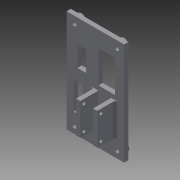
# Autodesk Inventor part: holder_board_basecam_simpleBCG_32bit_tiny
Saved by Autodesk Inventor 2015 SP1 (Build 190203100, 203)
## iProperties
Created: 2015-08-27
Part Number: holder_board_basecam_simpleBCG_32bit_tiny
Material: Generic
Document SubType Name: Modeling
Designer: Alexandre Cherpillod
Density: 1 g/cm^3
Appearance: Default
Author: Alexandre Cherpillod
Autodesk Inventor part; units mm, degrees
ref_plane "YZ Plane" through (0, 0, 0) normal (1, 0, 0) x (0, 1, 0)
ref_plane "XZ Plane" through (0, 0, 0) normal (0, 1, 0) x (-1, 0, 0)
ref_plane "XY Plane" through (0, 0, 0) normal (0, 0, 1) x (1, 0, 0)
sketch "Sketch1" plane through (0, 0, 0) normal (0, 1, 0) x (-1, 0, 0)
  circle A0 centre (0, 0) radius 2.4
  circle A1 centre (20, 0) radius 2.4
  circle A2 centre (20, -41.5) radius 2.4
  circle A3 centre (0, -41.5) radius 2.4
  dimension "d0" = 4.8
  dimension "d4" = 20
  dimension "d5" = 41.5
  constraints: 4 centre point, 3 equal radius, 1 coincident
  measures "d0" diameter of A0
  measures "d4" distance of point (0, 0) A1.centre
  measures "d5" distance of A2.centre A1.centre
extrude "Extrusion1" add sketch "Sketch1" along normal blind 1.5
sketch "Sketch2" plane through (0, 0, 0) normal (0, -1, 0) x (1, 0, 0)
  circle A0 centre (0, 0) radius 2.4 construction
  circle A1 centre (0, -41.5) radius 2.4 construction
  circle A2 centre (-20, -41.5) radius 2.4 construction
  circle A3 centre (-20, 0) radius 2.4 construction
  line L0 (3.492, 3.2394) -> (-23.508, 3.2394)
  line L1 (-23.508, 3.2394) -> (-23.508, -44.7606)
  line L2 (-23.508, -44.7606) -> (3.492, -44.7606)
  line L3 (3.492, -44.7606) -> (3.492, 3.2394)
  dimension "d8" = 27
  dimension "d9" = 48
  constraints: 8 end point, 2 parallel, 1 horizontal, 1 perpendicular
  measures "d8" distance of L0.start L0.end
  measures "d9" distance of L2.end L0.start
extrude "Extrusion2" add sketch "Sketch2" along normal blind 2
sketch "Sketch3" plane through (0, -2, 0) normal (0, -1, 0) x (1, 0, 0)
  circle A0 centre (0, 0) radius 2.4 construction
  circle A1 centre (0, -41.5) radius 2.4 construction
  circle A2 centre (-20, -41.5) radius 2.4 construction
  circle A3 centre (-20, 0) radius 2.4 construction
  line L0 (-8.5471, -21.5) -> (-10.5471, -21.5)
  line L1 (-10.5471, -21.5) -> (-10.5471, -36.5)
  line L2 (-10.5471, -36.5) -> (-8.5471, -36.5)
  line L3 (-8.5471, -36.5) -> (-8.5471, -21.5)
  line L4 (-0.5471, -21.5) -> (-2.5471, -21.5)
  line L5 (-2.5471, -21.5) -> (-2.5471, -36.5)
  line L6 (-2.5471, -36.5) -> (-0.5471, -36.5)
  line L7 (-0.5471, -36.5) -> (-0.5471, -21.5)
  line L8 (0, 0) -> (0, -41.5) construction
  dimension "d12" = 2
  dimension "d13" = 2
  dimension "d14" = 15
  dimension "d15" = 6
  dimension "d17" = 5
  constraints: 18 end point, 5 parallel, 2 horizontal, 2 perpendicular, 1 point on line, 1 vertical
  measures "d12" distance of L2.end L1.end
  measures "d13" distance of L6.end L5.end
  measures "d14" distance of L6.end L4.start
  measures "d15" distance between parallel lines of L3 L5
  measures "d17" distance from line of L8.end L6
extrude "Extrusion3" add sketch "Sketch3" along normal blind 8.5
sketch "Sketch4" plane through (-10.5471, -2, -36.5) normal (-1, 0, 0) x (0, 0, 1)
  line L0 (15, 0) -> (15, -8.5) construction
  line L1 (15, -6) -> (0, -6) construction
  line L2 (0, 0) -> (0, -8.5) construction
  circle A0 centre (13.1106, -6.75) radius 0.75
  circle A1 centre (1.8252, -6.75) radius 0.75
  line L3 (39.7394, 0) -> (-8.2606, 0) projected
  point P0 (36.5, 2)
  dimension "d21" = 1.5
  dimension "d22" = 0.75
  dimension "d23" = 1.5
  dimension "d24" = 0.75
  dimension "d25" = 6
  constraints: 2 centre point, 2 end point, 2 point on line, 1 horizontal
  measures "d21" diameter of A0
  measures "d22" distance from line of L1 A0.centre
  measures "d23" diameter of A1
  measures "d24" distance from line of L1 A1.centre
  measures "d25" distance between parallel lines of L3 L1
extrude "Extrusion4" cut sketch "Sketch4" against normal through all
sketch "Sketch6" plane through (0, -2, 0) normal (0, -1, 0) x (1, 0, 0)
  line L0 (-0.7166, -4.3244) -> (-8.5921, -4.3244)
  line L1 (-8.5921, -4.3244) -> (-8.5921, -19.4025)
  line L2 (-8.5921, -19.4025) -> (-0.7166, -19.4025)
  line L3 (-0.7166, -19.4025) -> (-0.7166, -4.3244)
  line L4 (-14.3515, -7.8111) -> (-18.4107, -7.8111)
  line L5 (-18.4107, -7.8111) -> (-18.4107, -17.2306)
  line L6 (-18.4107, -17.2306) -> (-14.3515, -17.2306)
  line L7 (-14.3515, -17.2306) -> (-14.3515, -7.8111)
  line L8 (-15.9648, -22.747) -> (-20.1801, -22.747)
  line L9 (-20.1801, -22.747) -> (-20.1801, -35.9136)
  line L10 (-20.1801, -35.9136) -> (-15.9648, -35.9136)
  line L11 (-15.9648, -35.9136) -> (-15.9648, -22.747)
  point P0 (0, 0)
  constraints: 24 end point, 6 parallel, 3 horizontal, 3 perpendicular
extrude "Extrusion6" cut sketch "Sketch6" against normal through all
hole "Hole1" at (0, 1.5, -41.5) direction (0, -1, 0) diameter 2.2 depth 8 tip angle 118
hole "Hole2" at (0, 1.5, 0) direction (0, -1, 0) diameter 2.2 depth 8 tip angle 118
hole "Hole3" at (-20, 1.5, -41.5) direction (0, -1, 0) diameter 2.2 depth 8 tip angle 118
hole "Hole4" at (-20, 1.5, 0) direction (0, -1, 0) diameter 2.2 depth 8 tip angle 118
fillet "Fillet1" radius 0.7 4 edges at (-17.6, 0, 0) (2.4, 0, 0) (2.4, 0, -41.5) (-17.6, 0, -41.5)
fillet "Fillet2" radius 1.3 2 edges at (-10.5471, -2, -29) (-0.5471, -2, -29)
body "Solid1"
